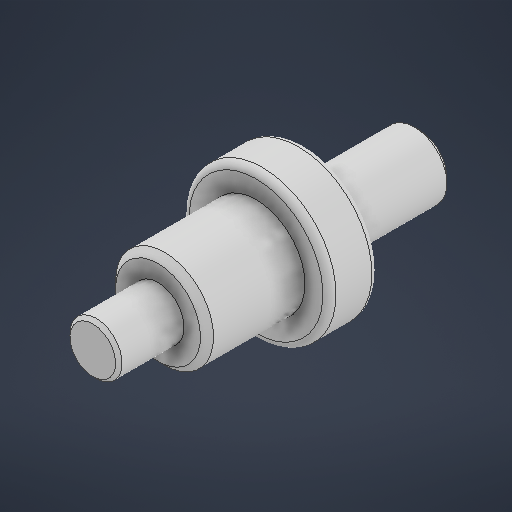
# Autodesk Inventor part: Part5
Saved by Autodesk Inventor 2026 (Build 300175050, 175E)
## iProperties
Created: 2026-03-26
Part Number: Part5
Material: Generic
Document SubType Name: Modeling
Designer: Administrator
Density: 1 g/cm^3
Appearance: Default
Author: Administrator
Autodesk Inventor part; units mm, degrees
ref_plane "YZ Plane" through (0, 0, 0) normal (1, 0, 0) x (0, 1, 0)
ref_plane "XZ Plane" through (0, 0, 0) normal (0, 1, 0) x (-1, 0, 0)
ref_plane "XY Plane" through (0, 0, 0) normal (0, 0, 1) x (1, 0, 0)
sketch "Sketch1" plane through (0, 0, 0) normal (1, 0, 0) x (0, 1, 0)
  line L0 (0, 0) -> (0, -100)
  line L1 (0, 0) -> (8, 0)
  line L2 (8, 0) -> (8, -20)
  line L3 (8, -20) -> (15, -20)
  line L4 (15, -20) -> (15, -50)
  line L5 (15, -50) -> (22.5, -50)
  line L6 (22.5, -50) -> (22.5, -65)
  line L7 (22.5, -65) -> (10, -65)
  line L8 (10, -65) -> (10, -100)
  line L9 (10, -100) -> (0, -100)
  dimension "d0" = 100
  dimension "d1" = 8
  dimension "d2" = 20
  dimension "d3" = 7
  dimension "d4" = 30
  dimension "d5" = 7.5
  dimension "d6" = 15
  dimension "d7" = 12.5
  constraints: 20 end point, 6 perpendicular, 2 horizontal, 2 vertical
  measures "d0" distance of L0.start L0.end
  measures "d1" distance of L0.start L1.end
  measures "d2" distance of L1.end L2.end
  measures "d3" distance of L2.end L3.end
  measures "d4" distance of L3.end L4.end
  measures "d5" distance of L4.end L5.end
  measures "d6" distance of L5.end L6.end
  measures "d7" distance of L6.end L7.end
revolve "Revolution1" add sketch "Sketch1" angle 360 about axis through (0, 0, 0) along (0, 0, -1)
chamfer "Chamfer1" distance 2 angle 45 1 edges at (0, -15, -20)
chamfer "Chamfer2" distance 1 angle 45 1 edges at (0, -8, 0)
fillet "Fillet1" radius 2 1 edges at (0, -22.5, -50)
fillet "Fillet2" radius 2 1 edges at (0, -22.5, -65)
fillet "Fillet3" radius 4 1 edges at (0, -10, -65)
chamfer "Chamfer3" distance 1.5 angle 45 1 edges at (0, -10, -100)
body "Solid1"
